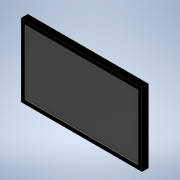
# Autodesk Inventor part: Monitor_21inch
Saved by Autodesk Inventor 2020 (Build 240168000, 168)
## iProperties
Created: 2021-07-08
Part Number: Monitor_21inch
Material: Generic
Document SubType Name: Modeling
Designer: Simon.Alvarez
Density: 1 g/cm^3
Appearance: Default
Author: Simon.Alvarez
Autodesk Inventor part; units mm, degrees
ref_plane "YZ Plane" through (0, 0, 0) normal (1, 0, 0) x (0, 1, 0)
ref_plane "XZ Plane" through (0, 0, 0) normal (0, 1, 0) x (-1, 0, 0)
sketch "Sketch1" plane through (0, 0, 0) normal (0, 0, 1) x (1, 0, 0)
  line L0 (-236.5, -142.5) -> (236.5, -142.5)
  line L1 (236.5, -142.5) -> (236.5, 142.5)
  line L2 (236.5, 142.5) -> (-236.5, 142.5)
  line L3 (-236.5, 142.5) -> (-236.5, -142.5)
  line L4 (-236.5, -142.5) -> (236.5, 142.5) construction
  line L5 (236.5, -142.5) -> (-236.5, 142.5) construction
  point P0 (0, 0)
  dimension "d0" = 473
  dimension "d1" = 285
  constraints: 12 end point, 2 midpoint, 2 parallel, 1 horizontal, 1 perpendicular
  measures "d0" distance of L1.end L2.end
  measures "d1" distance of L2.end L0.start
extrude "Extrusion1" add sketch "Sketch1" against normal blind 26
sketch "Sketch2" plane through (0, 0, -26) normal (0, 0, -1) x (-1, 0, 0)
  line L0 (-233.5, -139.5) -> (233.5, -139.5)
  line L1 (233.5, -139.5) -> (233.5, 139.5)
  line L2 (233.5, 139.5) -> (-233.5, 139.5)
  line L3 (-233.5, 139.5) -> (-233.5, -139.5)
  line L4 (-233.5, -139.5) -> (233.5, 139.5) construction
  line L5 (233.5, -139.5) -> (-233.5, 139.5) construction
  line L6 (236.5, 142.5) -> (-236.5, 142.5) projected
  line L7 (-236.5, 142.5) -> (-236.5, -142.5) projected
  point P0 (0, 0)
  dimension "d4" = 3
  dimension "d5" = 3
  constraints: 12 end point, 2 midpoint, 2 parallel, 1 horizontal, 1 perpendicular
  measures "d4" distance between parallel lines of L2 L6
  measures "d5" distance between parallel lines of L3 L7
ref_plane "Work Plane1" through (0, 0, -66) normal (0, 0, -1) x (-1, 0, 0)
sketch "Sketch4" plane through (0, 0, -66) normal (0, 0, -1) x (-1, 0, 0)
  line L0 (-190, -70) -> (190, -70)
  line L1 (190, -70) -> (190, 70)
  line L2 (190, 70) -> (-190, 70)
  line L3 (-190, 70) -> (-190, -70)
  line L4 (-190, -70) -> (190, 70) construction
  line L5 (190, -70) -> (-190, 70) construction
  point P0 (0, 0)
  dimension "d7" = 140
  dimension "d8" = 380
  constraints: 12 end point, 2 midpoint, 2 parallel, 1 horizontal, 1 perpendicular
  measures "d7" distance of L2.end L0.start
  measures "d8" distance of L1.end L2.end
loft "Loft1" add profiles "Sketch2", "Sketch4"
sketch "Sketch5" plane through (190, -70, -66) normal (0, 0, -1) x (-1, 0, 0)
  line L0 (140, 20) -> (240, 20)
  line L1 (240, 20) -> (240, 120)
  line L2 (240, 120) -> (140, 120)
  line L3 (140, 120) -> (140, 20)
  line L4 (140, 20) -> (240, 120) construction
  line L5 (240, 20) -> (140, 120) construction
  point P0 (190, 70)
  dimension "d13" = 100
  dimension "d14" = 100
  constraints: 12 end point, 4 coincident, 2 midpoint, 2 parallel, 1 horizontal, 1 perpendicular
  measures "d13" distance of L1.end L2.end
  measures "d14" distance of L2.end L0.start
hole "Hole1" at (50, 50, -66) at (-50, 50, -66) at (-50, -50, -66) at (50, -50, -66) direction (0, 0, 1) diameter 4.134 depth 15 tip angle 118 thread size "M5x0.8" class "6H" standard "ANSI Metric M Profile"
sketch "Sketch6" plane through (0, 0, 0) normal (0, 0, 1) x (1, 0, 0)
  line L0 (-221.5, -127.5) -> (221.5, -127.5)
  line L1 (221.5, -127.5) -> (221.5, 127.5)
  line L2 (221.5, 127.5) -> (-221.5, 127.5)
  line L3 (-221.5, 127.5) -> (-221.5, -127.5)
  line L4 (-221.5, -127.5) -> (221.5, 127.5) construction
  line L5 (221.5, -127.5) -> (-221.5, 127.5) construction
  line L6 (236.5, 142.5) -> (-236.5, 142.5) projected
  line L7 (-236.5, 142.5) -> (-236.5, -142.5) projected
  point P0 (0, 0)
  dimension "d22" = 15
  dimension "d23" = 15
  constraints: 12 end point, 2 midpoint, 2 parallel, 1 horizontal, 1 perpendicular
  measures "d22" distance between parallel lines of L2 L6
  measures "d23" distance between parallel lines of L7 L3
extrude "Extrusion2" cut sketch "Sketch6" against normal blind 4
body "Solid1"
